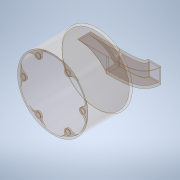
# Autodesk Inventor part: Dust Bin
Saved by Autodesk Inventor 2020 (Build 240168000, 168)
## iProperties
Created: 2020-03-28
Part Number: Dust Bin
Material: Generic
Document SubType Name: Modeling
Designer: pengpeng
Density: 1 g/cm^3
Appearance: Polycarbonate - Smoked
Author: pengpeng
Autodesk Inventor part; units mm, degrees
ref_plane "YZ Plane" through (0, 0, 0) normal (1, 0, 0) x (0, 1, 0)
sketch "Sketch1" plane through (0, 0, 0) normal (0, 0, 1) x (1, 0, 0)
  circle A0 centre (0, 0) radius 68
  dimension "d1" = 136
  constraints: 1 centre point
  measures "d1" diameter of A0
extrude "Extrusion1" add sketch "Sketch1" along normal blind 80
shell "Shell1" thickness 3 removed faces 1 at (13.6377, 7.7647, 0)
sketch "Sketch2" plane through (0, 0, 80) normal (0, 0, 1) x (1, 0, 0)
  circle A0 centre (0, 0) radius 32
  dimension "d5" = 64
  constraints: 1 centre point, 1 coincident
  measures "d5" diameter of A0
extrude "Extrusion2" cut sketch "Sketch2" against normal up to surface (3 mm away)
sketch "Sketch3" plane through (0, 0, 77) normal (0, 0, -1) x (-1, 0, 0)
  circle A0 centre (0, 0) radius 32 projected
  circle A1 centre (0, 0) radius 65 projected
  circle A2 centre (0, -40) radius 4.8
  line L0 (0, 0) -> (0, -56.282) construction
  line L1 (0, 0) -> (-47.9956, 27.7103) construction
  line L2 (0, 0) -> (60.1339, 34.7183) construction
  circle A3 centre (-34.641, 20) radius 4.8
  circle A4 centre (34.641, 20) radius 4.8
  dimension "d8" = 9.6
  dimension "d9" = 40
  dimension "d10" = 120
  dimension "d11" = 120
  dimension "d12" = 9.6
  dimension "d13" = 9.6
  dimension "d14" = 40
  dimension "d15" = 40
  constraints: 6 end point, 3 centre point, 2 point on line, 1 vertical
  measures "d8" diameter of A2
  measures "d9" distance of point (0, 0) A2.centre
  measures "d10" angle of L0 L1
  measures "d11" angle of L0 L2
  measures "d12" diameter of A3
  measures "d13" diameter of A4
  measures "d14" distance of point (0, 0) A4.centre
  measures "d15" distance of point (0, 0) A3.centre
extrude "Extrusion3" cut sketch "Sketch3" against normal blind 1.524 contours A2 | A3 | A4
ref_plane "Work Plane1" through (0, 0, 35) normal (0, 0, 1) x (1, 0, 0)
sketch "Sketch4" plane through (0, 0, 35) normal (0, 0, 1) x (1, 0, 0)
  circle A0 centre (0, 0) radius 68 projected
  circle A1 centre (0, 0) radius 68 projected
  line L0 (0, 68) -> (56.3915, 68)
  line L1 (56.3915, 68) -> (56.3915, 38)
  line L2 (56.3915, 38) -> (0, 38)
  line L3 (0, 38) -> (0, 68)
  dimension "d24" = 30
  constraints: 8 end point, 2 horizontal, 2 parallel, 1 perpendicular, 1 vertical alignment, 3 other
  measures "d24" distance between parallel lines of L2 L0
extrude "Extrusion4" add sketch "Sketch4" against normal blind 25 contours A0 L0 L1
sketch "Sketch6" plane through (56.3915, 38, 35) normal (1, 0, 0) x (0, 0, -1)
  line L0 (0, 0) -> (0, 30) projected
  line L1 (25, 0) -> (0, 0) projected
  line L2 (25, 30) -> (25, 0) projected
  line L3 (0, 30) -> (25, 30) projected
  line L4 (22, 27) -> (22, 3)
  line L5 (22, 3) -> (3, 3)
  line L6 (3, 3) -> (3, 27)
  line L7 (3, 27) -> (22, 27)
  point P0 (35, -38)
  dimension "d27" = 3
  constraints: 8 end point, 3 other
  measures "d27" distance between parallel lines of L3 L7
extrude "Extrusion5" cut sketch "Sketch6" against normal blind 56.391 contours L4 L5 L6 L7
ref_plane "Work Plane4" through (0, 68, 0) normal (0, 1, 0) x (-1, 0, 0)
sketch "Sketch9" plane through (56.3915, 38, 35) normal (1, 0, 0) x (0, 0, -1)
  line L0 (3, 3) -> (3, 27) projected
  line L1 (3, 27) -> (22, 27) projected
  line L2 (22, 27) -> (22, 3) projected
  line L3 (22, 3) -> (3, 3) projected
  line L4 (0, 0) -> (0, 30) projected
  line L5 (25, 0) -> (0, 0) projected
  line L6 (25, 30) -> (25, 0) projected
  line L7 (0, 30) -> (25, 30) projected
  point P0 (35, -38)
sketch "Sketch10" plane through (0, 68, 0) normal (0, 1, 0) x (-1, 0, 0)
  line L0 (-160.9388, 35) -> (106.1565, 35) projected
  line L1 (-56.3915, 35) -> (0, 35) projected
  line L2 (0, 0) -> (-96.3915, 0) construction
  line L3 (-68, 0) -> (-68, 80) projected
  line L4 (-56.3915, 35) -> (-91.3915, 35) construction
  line L5 (-91.3915, 35) -> (-126.3915, 35) construction
  line L6 (-126.3915, 35) -> (-126.3915, 0) construction
  spline S0 degree 3 poles (-56.3915, 35) (-91.3915, 35) (-126.3915, 35) (-126.3915, 0) knots 1 1 1 1 2 2 2 2
  line L7 (-126.3915, 0) -> (-126.3915, 60.9318) construction
  point P0 (-91.3915, 0)
  dimension "d113" = 70
  dimension "d114" = 35
  dimension "d115" = 35
  constraints: 4 end point, 2 horizontal, 1 coincident, 1 perpendicular, 1 point on line, 1 vertical, 3 other
  measures "d113" horizontal distance of L4.start L6.end
  measures "d114" distance of L4.start L4.end
  measures "d115" distance of L6.end L5.end
sweep "Sweep2" add profiles "Sketch9" path "Sketch10" path curves S0
sketch "Sketch11" plane through (0, 0, 77) normal (0, 0, -1) x (-1, 0, 0)
  circle A0 centre (-34.641, 20) radius 4.8 projected
  circle A1 centre (34.641, 20) radius 4.8 projected
  circle A2 centre (0, -40) radius 4.8 projected
  circle A3 centre (0, 0) radius 32 projected
  circle A4 centre (0, 0) radius 65 projected
  circle A5 centre (-34.641, 20) radius 6.3
  circle A6 centre (34.641, 20) radius 6.3
  circle A7 centre (0, -40) radius 6.3
  circle A8 centre (0, 0) radius 33.5
  line L0 (-36.0415, 26.1424) -> (-7.4468, 32.6618)
  line L1 (-40.6607, 18.1416) -> (-32.0094, -9.8818)
  line L2 (36.0415, 26.1424) -> (7.4468, 32.6618)
  line L3 (40.6607, 18.1416) -> (32.0094, -9.8818)
  line L4 (4.6192, -44.284) -> (24.5626, -22.78)
  line L5 (-4.6192, -44.284) -> (-24.5626, -22.78)
  circle A9 centre (-34.641, 20) radius 7.8
  line L6 (-42.0939, 17.6992) -> (-34.7194, -6.1884)
  circle A10 centre (34.641, 20) radius 7.8
  circle A11 centre (0, -40) radius 7.8
  line L7 (-36.3749, 27.6048) -> (-12.0004, 33.1621)
  line L8 (36.3749, 27.6048) -> (12.0004, 33.1621)
  line L9 (42.0939, 17.6992) -> (34.7194, -6.1884)
  line L10 (5.7191, -45.304) -> (22.7191, -26.9737)
  line L11 (-5.7191, -45.304) -> (-22.7191, -26.9737)
  line L12 (-34.7194, -6.1884) -> (-33.2862, -5.746)
  line L13 (-22.7191, -26.9737) -> (-21.6192, -25.9537)
  line L14 (12.0004, 33.1621) -> (11.6669, 31.6997)
  line L15 (34.7194, -6.1884) -> (33.2862, -5.746)
  line L16 (22.7191, -26.9737) -> (21.6192, -25.9537)
  line L17 (-12.0004, 33.1621) -> (-11.6669, 31.6997)
  dimension "d39" = 1.5
  dimension "d40" = 1.5
  dimension "d41" = 1.5
  dimension "d42" = 1.5
  dimension "d43" = 1.5
  dimension "d44" = 1.5
  dimension "d45" = 1.5
  dimension "d46" = 25
  dimension "d47" = 25
  dimension "d48" = 25
  dimension "d49" = 25
  dimension "d50" = 25
  dimension "d51" = 25
  constraints: 36 end point, 18 point on circle, 18 tangent, 7 centre point, 6 parallel, 6 perpendicular, 6 point on line
  measures "d39" radial gap between concentric circles of A0 A5
  measures "d40" radial gap between concentric circles of A1 A6
  measures "d41" radial gap between concentric circles of A2 A7
  measures "d42" radial gap between concentric circles of A8 A3
  measures "d43" radial gap between concentric circles of A5 A9
  measures "d44" radial gap between concentric circles of A6 A10
  measures "d45" radial gap between concentric circles of A7 A11
  measures "d46" distance of L6.start L6.end
  measures "d47" distance of L7.start L7.end
  measures "d48" distance of L8.start L8.end
  measures "d49" distance of L9.start L9.end
  measures "d50" distance of L10.start L10.end
  measures "d51" distance of L11.start L11.end
extrude "Extrusion6" add sketch "Sketch11" along normal blind 1.5 contours A5 L1 A9 L0 | A9 L7 L17 L0 | L1 L12 L6 A9 | L14 L8 A10 L2 | L5 A11 L11 L13 | A10 L3 A6 L2 | L5 A7 L4 A11 | A10 L9 L15 L3 | L16 L10 A11 L4
sketch "Sketch14" plane through (0, 0, 80) normal (0, 0, 1) x (1, 0, 0)
  circle A0 centre (0, 0) radius 32 projected
  line L0 (0, 0) -> (0, 28.9416) construction
  circle A1 centre (0, 41) radius 3
  line L1 (0, 0) -> (-25.0642, -14.4708) construction
  line L2 (0, 0) -> (25.0642, -14.4708) construction
  point P0 (-35.507, -20.5)
  point P1 (-35.507, -20.5)
  point P2 (35.507, -20.5)
  point P3 (35.507, -20.5)
  dimension "d98" = 6
  dimension "d99" = 41
  dimension "d102" = 360
  constraints: 6 end point, 3 coincident, 3 point on line, 1 centre point, 1 vertical, 16 other
  measures "d98" diameter of A1
  measures "d99" distance of point (0, 0) A1.centre
hole "Hole1" at (0, 41, 80) at (-35.507, -20.5, 80) at (35.507, -20.5, 80) direction (0, 0, -1) diameter 6 end through all
sketch "Sketch16" plane through (0, 0, 0) normal (0, 0, -1) x (-1, 0, 0)
  circle A0 centre (0, 0) radius 68 projected
extrude "Extrusion9" add sketch "Sketch16" along normal blind 3
sketch "Sketch17" plane through (0, 0, 75.5) normal (0, 0, -1) x (-1, 0, 0)
  circle A0 centre (0, 0) radius 65 projected
extrude "Extrusion10" cut sketch "Sketch17" against normal up to surface (4.5 mm away)
sketch "Sketch18" plane through (0, 0, 80) normal (0, 0, 1) x (1, 0, 0)
  circle A0 centre (0, 0) radius 65 projected
  circle A1 centre (0, 0) radius 68 projected
  line L0 (0, 0) -> (-83.6751, 0) construction
  circle A2 centre (-57.5, 0) radius 4.8
  circle A3 centre (-57.5, 0) radius 6.3
  circle A4 centre (-52.744, -15.5907) radius 10
  circle A5 centre (-52.744, 15.5907) radius 10
  circle A6 centre (0, 0) radius 65 projected
  circle A7 centre (-28.75, -49.7965) radius 6.3
  circle A8 centre (-28.75, -49.7965) radius 4.8
  circle A9 centre (-39.874, -37.8823) radius 10
  circle A10 centre (-12.87, -53.473) radius 10
  circle A11 centre (28.75, -49.7965) radius 6.3
  circle A12 centre (28.75, -49.7965) radius 4.8
  circle A13 centre (12.87, -53.473) radius 10
  circle A14 centre (39.874, -37.8823) radius 10
  circle A15 centre (57.5, 0) radius 6.3
  circle A16 centre (57.5, 0) radius 4.8
  circle A17 centre (52.744, -15.5907) radius 10
  circle A18 centre (52.744, 15.5907) radius 10
  circle A19 centre (28.75, 49.7965) radius 6.3
  circle A20 centre (28.75, 49.7965) radius 4.8
  circle A21 centre (39.874, 37.8823) radius 10
  circle A22 centre (12.87, 53.473) radius 10
  circle A23 centre (-28.75, 49.7965) radius 6.3
  circle A24 centre (-28.75, 49.7965) radius 4.8
  circle A25 centre (-12.87, 53.473) radius 10
  circle A26 centre (-39.874, 37.8823) radius 10
  point P0 (-55.6618, 6.0259)
  point P1 (-62.3338, 18.4254)
  point P2 (-47.1238, 44.77)
  point P3 (-33.0494, 45.1916)
  point P4 (-22.6123, 51.2175)
  point P5 (-15.2101, 63.1954)
  point P6 (15.2101, 63.1954)
  point P7 (22.6123, 51.2175)
  point P8 (33.0494, 45.1916)
  point P9 (47.1238, 44.77)
  point P10 (62.3338, 18.4254)
  point P11 (55.6618, 6.0259)
  point P12 (55.6618, -6.0259)
  point P13 (62.3338, -18.4254)
  point P14 (47.1238, -44.77)
  point P15 (33.0494, -45.1916)
  point P16 (22.6123, -51.2175)
  point P17 (15.2101, -63.1954)
  point P18 (-15.2101, -63.1954)
  point P19 (-22.6123, -51.2175)
  point P20 (-33.0494, -45.1916)
  point P21 (-47.1238, -44.77)
  point P22 (-62.3338, -18.4254)
  point P23 (-55.6618, -6.0259)
  dimension "d118" = 9.6
  dimension "d119" = 57.5
  dimension "d120" = 1.5
  dimension "d121" = 20
  dimension "d122" = 20
  dimension "d125" = 360
  constraints: 24 centre point, 4 tangent, 2 end point, 1 horizontal, 1 point on line, 43 other
  measures "d118" diameter of A2
  measures "d119" distance of point (0, 0) A2.centre
  measures "d120" radial gap between concentric circles of A2 A3
  measures "d121" diameter of A4
  measures "d122" diameter of A5
extrude "Extrusion11" add sketch "Sketch18" along normal blind 3 contours A0 A17 A15 A18 | A21 A19 A22 A0 | A15 | A0 A13 A11 A14 | A19 | A11 | A25 A23 A26 A0 | A0 A9 A7 A10 | A23 | A7 | A5 A3 A4 A0 | A3 | A1 | A2 | A8 | A12 | A16 | A20 | A24
sketch "Sketch19" plane through (0, 0, 83) normal (0, 0, 1) x (1, 0, 0)
  line L0 (0, 0) -> (-55.7634, 0) construction
  circle A0 centre (0, 0) radius 68 projected
  circle A1 centre (-57.5, 0) radius 4.8
  circle A2 centre (-28.75, -49.7965) radius 4.8
  circle A3 centre (28.75, -49.7965) radius 4.8
  circle A4 centre (57.5, 0) radius 4.8
  circle A5 centre (28.75, 49.7965) radius 4.8
  circle A6 centre (-28.75, 49.7965) radius 4.8
  dimension "d129" = 9.6
  dimension "d130" = 57.5
  dimension "d133" = 360
  constraints: 6 centre point, 2 end point, 1 horizontal, 1 point on line, 13 other
  measures "d129" diameter of A1
  measures "d130" distance of L0.start A1.centre
extrude "Extrusion12" cut sketch "Sketch19" against normal blind 1.524 contours A1 | A2 | A3 | A4 | A5 | A6
equation "\"d11\" = d10"
equation "\"d12\" = d8"
equation "\"d13\" = d8"
equation "\"d14\" = d9"
equation "\"d15\" = d9"
equation "\"d40\" = d39"
equation "\"d41\" = d39"
equation "\"d42\" = d39"
equation "\"d44\" = d43"
equation "\"d45\" = d41"
equation "\"d47\" = d46"
equation "\"d48\" = d47"
equation "\"d49\" = d48"
equation "\"d50\" = d49"
equation "\"d51\" = d50"
equation "\"d122\" = d121"
body "Solid1"
